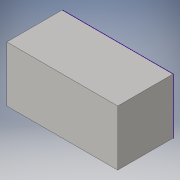
# Autodesk Inventor part: IED7_Sun_PuzzleCubePink
Saved by Autodesk Inventor 2016 (Build 200138000, 138)
## iProperties
Created: 2017-09-29
Part Number: IED7_Sun_PuzzleCubePink
Material: Generic
Document SubType Name: Sheet Metal
Designer: sun01147
Density: 1 g/cm^3
Sheet Metal Rule: Default
Appearance: Default
Author: sun01147
Autodesk Inventor part; units mm, degrees
ref_plane "YZ Plane" through (0, 0, 0) normal (1, 0, 0) x (0, 1, 0)
ref_plane "XZ Plane" through (0, 0, 0) normal (0, 1, 0) x (-1, 0, 0)
ref_plane "XY Plane" through (0, 0, 0) normal (0, 0, 1) x (1, 0, 0)
sketch "Sketch1" plane through (0, 0, 0) normal (0, 0, 1) x (1, 0, 0)
  line L0 (0, 19.05) -> (0, 0)
  line L1 (0, 19.05) -> (38.1, 19.05)
  line L2 (38.1, 19.05) -> (38.1, 0)
  line L3 (38.1, 0) -> (0, 0)
  line L4 (0, 19.05) -> (19.05, 19.05)
  dimension "d0" = 19.05
  dimension "d1" = 38.1
  constraints: 10 end point, 2 vertical, 1 horizontal, 1 midpoint, 1 perpendicular
  measures "d0" distance of L0.start L0.end
  measures "d1" distance of L0.start L1.end
extrude "Extrusion1" add sketch "Sketch1" against normal blind 19.05
sketch "Sketch2" plane through (0, 0, -19.05) normal (0, 0, -1) x (-1, 0, 0)
  line L0 (0, 19.05) -> (-38.1, 19.05) projected
  line L1 (-19.05, 19.05) -> (-19.05, 0)
  line L2 (-38.1, 0) -> (0, 0) projected
  line L3 (-38.1, 19.05) -> (-38.1, 0) projected
  line L4 (-38.1, 19.05) -> (-38.1, 0)
  line L5 (0, 0) -> (0, 19.05) projected
  line L6 (-38.1, 0) -> (0, 0)
  line L7 (-38.1, 19.05) -> (0, 19.05)
  line L8 (0, 19.05) -> (0, 0)
  constraints: 10 end point, 3 collinear, 2 midpoint, 1 perpendicular
equation "\"BendRadius\" = Thickness"
equation "\"BendReliefWidth\" = Thickness"
equation "\"BendReliefDepth\" = 0.5 * Thickness"
equation "\"CornerReliefSize\" = 4 * Thickness"
equation "\"MinimumRemnant\" = 2 * Thickness"
equation "\"TransitionRadius\" = BendRadius"
equation "\"JacobiRadiusSize\" = BendRadius"
equation "\"GapSize\" = Thickness"
equation "\"Thickness\" = 3.048"
body "Solid1"
